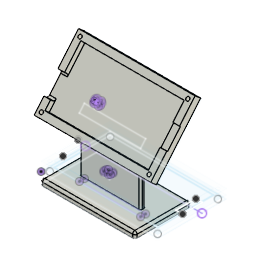
Kurokku case (Autodesk Fusion 360 design; units mm, degrees)
part number: 2026-06-15-00-16-35-276
Autodesk Fusion 360 part; units mm, degrees
sketch "Sketch1" plane through (0, 0, 0) normal (0, 0, 1) x (1, 0, 0)
  line L0 (0, 0) -> (105.33, 0)
  line L1 (105.33, 0) -> (105.33, 62.37)
  line L2 (105.33, 62.37) -> (0, 62.37)
  line L3 (0, 62.37) -> (0, 0)
  circle A0 centre (4, 58.37) radius 1.6
  circle A1 centre (101.33, 58.37) radius 1.6
  circle A2 centre (4, 4) radius 1.6
  circle A3 centre (101.33, 4) radius 1.6
  line L4 (31, 28.87) -> (37, 28.87)
  line L5 (37, 28.87) -> (37, 24.87)
  line L6 (37, 24.87) -> (31, 24.87)
  line L7 (31, 24.87) -> (31, 28.87)
  dimension "d1" = 105.33
  dimension "d2" = 62.37
  dimension "d3" = 3.2
  dimension "d4" = 4
  dimension "d5" = 4
  dimension "d6" = 3.2
  dimension "d7" = 4
  dimension "d8" = 4
  dimension "d9" = 3.2
  dimension "d10" = 4
  dimension "d11" = 4
  dimension "d12" = 3.2
  dimension "d13" = 4
  dimension "d14" = 4
  dimension "d38" = 6
  dimension "d39" = 4
  dimension "d40" = 31
  dimension "d41" = 33.5
  constraint horizontal L0
  constraint vertical L1
  constraint horizontal L2
  constraint vertical L3
  constraint coincident L0.start L3.end
  constraint horizontal L4
  constraint vertical L5
  constraint horizontal L6
  constraint vertical L7
  measures "d1" distance of L0.start L0.end
  measures "d2" distance of L0.start L2.end
  measures "d3" diameter of A0
  measures "d4" horizontal distance of L2.end A0.centre
  measures "d5" vertical distance of L2.end A0.centre
  measures "d6" diameter of A1
  measures "d7" horizontal distance of L1.end A1.centre
  measures "d8" vertical distance of L1.end A1.centre
  measures "d9" diameter of A2
  measures "d10" horizontal distance of L0.start A2.centre
  measures "d11" vertical distance of L0.start A2.centre
  measures "d12" diameter of A3
  measures "d13" horizontal distance of L0.end A3.centre
  measures "d14" vertical distance of L0.end A3.centre
  measures "d38" distance of L4.start L4.end
  measures "d39" distance of L4.start L6.end
  measures "d40" distance of L3 L7
  measures "d41" distance of L2 L4
extrude "Extrude1" add sketch "Sketch1" along normal blind 3.2 makes body 1
fillet "Fillet1" radius 1 4 edges at (37, 24.87, 1.6) (31, 24.87, 1.6) (31, 28.87, 1.6) (37, 28.87, 1.6) on bodies 1
sketch "Sketch2" plane through (0, 0, 3.2) normal (0, 0, 1) x (-1, 0, 0)
  circle A0 centre (-4, -58.37) radius 1.6
  circle A1 centre (-4, -4) radius 1.6
  circle A2 centre (-101.33, -58.37) radius 1.6
  circle A3 centre (-101.33, -4) radius 1.6
  line L0 (0, -62.37) -> (0, 0)
  line L1 (0, 0) -> (-105.33, 0)
  line L2 (-105.33, 0) -> (-105.33, -62.37)
  line L3 (-105.33, -62.37) -> (0, -62.37)
  line L4 (-36, -24.87) -> (-32, -24.87)
  line L5 (-31, -25.87) -> (-31, -27.87)
  line L6 (-32, -28.87) -> (-36, -28.87)
  line L7 (-37, -27.87) -> (-37, -25.87)
  arc A4 (-31, -25.87) -> (-32, -24.87) centre (-32, -25.87) ccw
  arc A5 (-32, -28.87) -> (-31, -27.87) centre (-32, -27.87) ccw
  arc A6 (-37, -27.87) -> (-36, -28.87) centre (-36, -27.87) ccw
  arc A7 (-36, -24.87) -> (-37, -25.87) centre (-36, -25.87) ccw
  line L8 (-99.33, -6) -> (-6, -6)
  line L9 (-6, -6) -> (-6, -56.37)
  line L10 (-6, -56.37) -> (-99.33, -56.37)
  line L11 (-99.33, -56.37) -> (-99.33, -6)
  dimension "d55" = 6
  dimension "d56" = 6
  dimension "d57" = 6
  dimension "d58" = 6
  constraint horizontal L8
  constraint vertical L9
  constraint horizontal L10
  constraint vertical L11
  measures "d55" distance of L1 L8
  measures "d56" distance of L2 L11
  measures "d57" distance of L3 L10
  measures "d58" distance of L0 L9
extrude "Extrude2" add sketch "Sketch2" along normal blind 5 contours L0 L1 L2 L3 bodies 1
sketch "Sketch8" plane through (0, 0, 8.2) normal (0, 0, 1) x (-1, 0, 0)
  circle A0 centre (-4, -58.37) radius 1.6
  circle A1 centre (-101.33, -4) radius 1.6
  line L0 (-6, -56.37) -> (-99.33, -56.37)
  line L1 (-99.33, -56.37) -> (-99.33, -6)
  line L2 (-99.33, -6) -> (-6, -6)
  line L3 (-6, -6) -> (-6, -56.37)
  circle A2 centre (-101.33, -58.37) radius 1.6
  circle A3 centre (-4, -4) radius 1.6
  line L4 (-105.33, -62.37) -> (0, -62.37)
  line L5 (0, -62.37) -> (0, 0)
  line L6 (0, 0) -> (-105.33, 0)
  line L7 (-105.33, 0) -> (-105.33, -62.37)
  line L8 (-99.33, -40.525) -> (-105.33, -40.525)
  line L9 (-105.33, -40.525) -> (-105.33, -22.525)
  line L10 (-105.33, -22.525) -> (-99.33, -22.525)
  line L11 (-99.33, -22.525) -> (-99.33, -40.525)
  line L12 (0, -33.47) -> (-6, -33.47)
  line L13 (-6, -33.47) -> (-6, -13.82)
  line L14 (-6, -13.82) -> (0, -13.82)
  line L15 (0, -13.82) -> (0, -33.47)
  dimension "d63" = 18
  dimension "d64" = 21.845
  dimension "d65" = 19.65
  dimension "d66" = 28.9
  constraint horizontal L8
  constraint vertical L9
  constraint horizontal L10
  constraint vertical L11
  constraint coincident L7 L9.end
  constraint coincident L1 L8.start
  constraint horizontal L12
  constraint vertical L13
  constraint horizontal L14
  constraint vertical L15
  constraint coincident L3 L13.end
  constraint coincident L5 L12.start
  measures "d63" distance of L8 L10
  measures "d64" distance of L4 L8
  measures "d65" distance of L12 L14
  measures "d66" distance of L4 L12
extrude "Extrude6" cut sketch "Sketch8" against normal blind 1 contours L0 L1 L2 L3 L11 L13 | L1 L7 L8 L9 L10 L11 bodies 1
extrude "Extrude7" cut sketch "Sketch8" against normal blind 5 contours L3 L5 L12 L13 L14 L15 bodies 1
move_body "Move1" bodies 1 to x (1, 0, 0) y (0, 0.642788, 0.766044) z (0, -0.766044, 0.642788) at (0, 0, 42)
sketch "Sketch4" plane through (0, -20.681, 17.3534) normal (0, 0.766044, -0.642788) x (-1, 0, 0)
  circle A0 centre (-101.33, 90.5439) radius 1.6
  circle A1 centre (-101.33, 36.1739) radius 1.6
  circle A2 centre (-4, 90.5439) radius 1.6
  circle A3 centre (-4, 36.1739) radius 1.6
  line L0 (0, 32.1739) -> (0, 94.5439)
  line L1 (0, 94.5439) -> (-105.33, 94.5439)
  line L2 (-105.33, 94.5439) -> (-105.33, 32.1739)
  line L3 (-105.33, 32.1739) -> (0, 32.1739)
  line L4 (-80.33, 54.1739) -> (-25, 54.1739)
  line L5 (-25, 54.1739) -> (-25, 47.1739)
  line L6 (-25, 47.1739) -> (-80.33, 47.1739)
  line L7 (-80.33, 47.1739) -> (-80.33, 54.1739)
  line L8 (-32, 57.0439) -> (-36, 57.0439)
  line L9 (-37, 58.0439) -> (-37, 60.0439)
  line L10 (-36, 61.0439) -> (-32, 61.0439)
  line L11 (-31, 60.0439) -> (-31, 58.0439)
  arc A4 (-37, 58.0439) -> (-36, 57.0439) centre (-36, 58.0439) ccw
  arc A5 (-36, 61.0439) -> (-37, 60.0439) centre (-36, 60.0439) ccw
  arc A6 (-31, 60.0439) -> (-32, 61.0439) centre (-32, 60.0439) ccw
  arc A7 (-32, 57.0439) -> (-31, 58.0439) centre (-32, 58.0439) ccw
  dimension "d29" = 55.33
  dimension "d30" = 25
  dimension "d31" = 15
  dimension "d32" = 7
  constraint horizontal L4
  constraint vertical L5
  constraint horizontal L6
  constraint vertical L7
  measures "d29" distance of L4.start L4.end
  measures "d30" distance of L2 L7
  measures "d31" distance of L3 L6
  measures "d32" distance of L4 L6
sketch "Sketch6" plane through (0, 0, 0) normal (0, 0, 1) x (1, 0, 0)
  line L0 (95.33, -10.6082) -> (10, -10.6082)
  line L1 (10, -10.6082) -> (10, 40.0908)
  line L2 (10, 40.0908) -> (95.33, 40.0908)
  line L3 (95.33, 40.0908) -> (95.33, -10.6082)
  line L4 (80.33, 14.1413) -> (25, 14.1413)
  line L5 (25, 9.6418) -> (80.33, 9.6418)
  line L6 (80.33, 9.6418) -> (80.33, 14.1413)
  line L7 (25, 14.1413) -> (25, 9.6418)
  line L8 (0, 40.0907) -> (105.33, 40.0907)
  dimension "d35" = 85.33
  dimension "d44" = 20.25
  dimension "d45" = 15
  dimension "d48" = 50.699
  constraint horizontal L0
  constraint vertical L1
  constraint horizontal L2
  constraint vertical L3
  measures "d35" distance of L0.start L0.end
  measures "d44" distance of L0 L5
  measures "d45" distance of L1 L7
  measures "d48" distance of L0 L2
extrude "Extrude5" add sketch "Sketch6" along normal blind 5 separate body makes body 2
loft "Loft2" add profiles "Sketch6", "Sketch4" section 1 contours L4 L5 L6 L7 section 2 contours L4 L5 L6 L7 bodies 1 2
fillet "Fillet2" radius 1.5 4 edges at (80.33, 14.1413, 31.9265) (80.33, 9.6418, 29.2453) (25, 14.1413, 31.9265) (25, 9.6418, 29.2453) on bodies 1
fillet "Fillet3" radius 2 8 edges at (52.665, -10.6082, 5) (95.33, -10.6082, 2.5) (95.33, 14.7413, 5) (95.33, 40.0908, 2.5) (52.665, 40.0908, 5) (10, 40.0908, 2.5) (10, 14.7413, 5) (10, -10.6082, 2.5) on bodies 1 2
fillet "Fillet4" radius 1.5 4 edges at (105.33, 20.0453, 65.8891) (52.665, 40.0907, 89.7782) (52.665, 0, 42) (0, 20.0453, 65.8891) on bodies 1
fillet "Fillet5" radius 2 2 edges at (3, 19.0628, 69.6964) (3, 6.432, 54.6437) on bodies 1
equation "d44 = ( ( 45 - 4.5 ) / 2 ) * 1 mm"
equation "d45 = ( ( 85.33 - 55.33 ) / 2 ) * 1 mm"
equation "d64 = 25 mm - 2.5 mm - ( ( ( 18 - 16.69 ) / 2 ) * 1 mm )"
